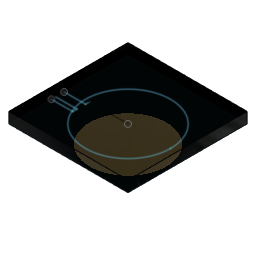
DS3231_PI v1 (Autodesk Fusion 360 design; units mm, degrees)
Autodesk Fusion 360 part; units mm, degrees
sketch "Esquisse1" plane through (0, 0, 0) normal (0, 0, 1) x (1, 0, 0)
  line L0 (0, 140) -> (14, 140)
  line L1 (14, 140) -> (14, 126)
  line L2 (14, 126) -> (0, 126)
  line L3 (0, 126) -> (0, 140)
  dimension "d3" = 14
  dimension "d4" = 14
  constraint horizontal L0
  constraint vertical L1
  constraint horizontal L2
  constraint vertical L3
  measures "d3" distance of L0 L2
  measures "d4" distance of L0.start L0.end
extrude "Extrusion1" add sketch "Esquisse1" along normal blind 1.27 makes body 1
sketch "Esquisse2" plane through (0, 0, 0) normal (0, 0, -1) x (1, 0, 0)
  line L0 (14, -126) -> (0, -126)
  line L1 (0, -126) -> (0, -140)
  line L2 (0, -140) -> (14, -140)
  line L3 (14, -140) -> (14, -126)
  circle A0 centre (7, -133) radius 5
  line L4 (0, -133) -> (7, -133)
  line L5 (0, -131) -> (2.5, -131)
  line L6 (2.5, -131) -> (2.5, -131.5)
  line L7 (2.5, -131.5) -> (0, -131.5)
  line L8 (0, -131.5) -> (0, -131)
  line L9 (0, -132.5) -> (2.5, -132.5)
  line L10 (2.5, -132.5) -> (2.5, -133)
  line L11 (2.5, -133) -> (0, -133)
  line L12 (0, -133) -> (0, -132.5)
  dimension "d11" = 10
  constraint horizontal L4
  constraint midpoint L1 L4.start
  constraint coincident A0.centre L4
  constraint coincident A0.centre L4.end
  constraint horizontal L5
  constraint vertical L6
  constraint horizontal L7
  constraint vertical L8
  constraint coincident L1 L5.start
  constraint horizontal L9
  constraint vertical L10
  constraint horizontal L11
  constraint vertical L12
  constraint coincident L4 L10.end
  constraint coincident L1 L9.start
  measures "d11" diameter of A0
extrude "Extrusion2" add sketch "Esquisse2" along normal blind 2 separate body contours A0 L5 L6 L7 | A0 L4 L5 L6 L7 L9 L10 L11 | A0 L4 L9 L10 L11 makes body 2
fillet "Congé1" radius 0.5 2 edges at (2.3384, 134.8081, -2) (2.3384, 134.8081, 0) on bodies 2
move_body "Déplacer2" bodies 2 to x (1, 0, 0) y (0, 1, 0) z (0, 0, 1) at (0, 0, -0.1)
extrude "Extrusion4" add sketch "Esquisse2" along normal blind 0.1 separate body contours L1 A0 L5 L7 L8 | L1 A0 L4 L9 L11 L12 makes body 3 at (0.7434, 131.3333, 0) makes body 4 at (0.6676, 132.7777, 0)
named bodies: "PCB", "Battery", "Connector1", "Connector2"
